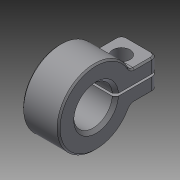
# Autodesk Inventor part: pipeClap
Saved by Autodesk Inventor 2014 SP1 (Build 180222100, 222)
## iProperties
Created: 2014-11-11
Part Number: pipeClap
Material: Generic
Document SubType Name: Modeling
Designer: rawrdong
Density: 1 g/cm^3
Appearance: Default
Author: rawrdong
Autodesk Inventor part; units mm, degrees
ref_plane "YZ Plane" through (0, 0, 0) normal (1, 0, 0) x (0, 1, 0)
ref_plane "XZ Plane" through (0, 0, 0) normal (0, 1, 0) x (-1, 0, 0)
ref_plane "XY Plane" through (0, 0, 0) normal (0, 0, 1) x (1, 0, 0)
sketch "Sketch1" plane through (0, 0, 0) normal (1, 0, 0) x (0, 1, 0)
  line L0 (0, 8.645) -> (0, -8.645) projected
  line L1 (-9.4444, 0) -> (13.4411, 0) projected
  circle A0 centre (0, 0) radius 6.175
  circle A1 centre (0, 0) radius 3.175
  line L2 (3.1687, -0.2) -> (6.1718, -0.2)
  line L3 (3.1687, 0.2) -> (6.1718, 0.2)
  line L4 (6.1718, 0.2) -> (10.1718, 0.2)
  line L5 (10.1718, 0.2) -> (10.1718, 2.45)
  line L6 (10.1718, 2.45) -> (5.6682, 2.45)
  line L7 (6.1718, -0.2) -> (10.1718, -0.2)
  line L8 (10.1718, -0.2) -> (10.1718, -2.45)
  line L9 (10.1718, -2.45) -> (5.6682, -2.45)
  dimension "d0" = 6.35
  dimension "d1" = 3
  dimension "d2" = 0.2
  dimension "d3" = 4
  dimension "d4" = 2.25
  constraints: 16 end point, 7 point on circle, 4 parallel, 2 centre point, 2 coincident, 2 perpendicular, 1 collinear, 1 point on line, 3 other
  measures "d0" diameter of A1
  measures "d1" radial gap between concentric circles of A0 A1
  measures "d2" distance between parallel lines of L3 L1
  measures "d3" distance of L7.start L7.end
  measures "d4" distance of L7.end L8.end
extrude "Extrusion1" add sketch "Sketch1" along normal blind 6 contours A0 L3 A1 L0 | L0 A1 L1 A0 | L6 L5 L4 A0 | L1 A1 L0 A0 | L0 A1 L2 A0 | A0 L7 L8 L9
sketch "Sketch2" plane through (0, 5.6682, -2.45) normal (0, 0, -1) x (-1, 0, 0)
  line L0 (0, 4.5036) -> (-6, 4.5036) projected
  circle A0 centre (-3, 1.5) radius 1.5
  circle A1 centre (-3, 1.5) radius 2.6 construction
  line L1 (0, 0) -> (-6, 0) projected
  point P0 (0, -5.6682)
  point P1 (-3, 4.5036)
  dimension "d8" = 3
  dimension "d24" = 5.2
  constraints: 2 centre point, 1 coincident, 1 midpoint, 1 tangent, 1 vertical alignment
  measures "d8" diameter of A0
  measures "d24" diameter of A1
extrude "Extrusion2" cut sketch "Sketch2" against normal up to surface (2.25 mm away)
sketch "Sketch4" plane through (0, 5.6682, 2.45) normal (0, 0, 1) x (1, 0, 0)
  circle A0 centre (3, 1.5) radius 1.5 projected
  circle A1 centre (3, 1.5) radius 1.5 projected
  circle A2 centre (3, 1.5) radius 1.425
  point P0 (0, -5.6682)
  point P1 (3, 0)
  dimension "d14" = 2.85
  constraints: 1 centre point, 1 coincident, 1 vertical alignment
  measures "d14" diameter of A2
extrude "Extrusion4" cut sketch "Sketch4" against normal through all contours A2
fillet "Fillet2" radius 1 7 edges at (6, 10.1718, 1.325) (3, 5.6682, 2.45) (0, 10.1718, 1.325) (0, 10.1718, -1.325) (6, 10.1718, -1.325) (1.5, 5.6682, -2.45) (4.5, 5.6682, -2.45)
chamfer "Chamfer1" distance 0.5 angle 45 2 edges at (6, -3.175, 0) (0, -3.175, 0)
sketch "Sketch5" plane through (0, 6.2911, -2.45) normal (0, 0, -1) x (-1, 0, 0)
  arc A0 (-1.7831, 0) -> (-4.2169, 0) centre (-3, 0.8771) ccw projected
  circle A1 centre (-3, 0.8771) radius 2.7
  circle A2 centre (-3, 0.8771) radius 1.5
  point P0 (0, -6.2911)
  dimension "d25" = 5.4
  constraints: 2 centre point, 2 coincident, 1 concentric
  measures "d25" diameter of A1
extrude "Extrusion5" cut sketch "Sketch5" along normal through all contours A2 A0 | A1
chamfer "Chamfer2" distance 0.25 angle 45 16 edges at (6, -6.175, 0) (6, 9.1718, -1.325) (6, 7.7314, -2.45) (5.7071, 9.8789, -2.45) (3, 10.1718, -2.45) (0.2929, 9.8789, -2.45) (0, 7.7314, -2.45) (0, 9.1718, -1.325) (0, -6.175, 0) (0, 9.1718, 1.325) (0, 7.7314, 2.45) (0.2929, 9.8789, 2.45) (3, 10.1718, 2.45) (5.7071, 9.8789, 2.45) (6, 7.7314, 2.45) (6, 9.1718, 1.325)
sketch "Sketch3" plane through (0, 5.6682, 2.45) normal (0, 0, 1) x (1, 0, 0)
  circle A0 centre (2.5, 3.2518) radius 1.5 projected
  circle A1 centre (2.5, 3.2518) radius 1.5 projected
  line L0 (4.3187, 6.4018) -> (6.1373, 3.2518)
  line L1 (6.1373, 3.2518) -> (4.3187, 0.1018)
  line L2 (4.3187, 0.1018) -> (0.6813, 0.1018)
  line L3 (0.6813, 0.1018) -> (-1.1373, 3.2518)
  line L4 (-1.1373, 3.2518) -> (0.6813, 6.4018)
  line L5 (0.6813, 6.4018) -> (4.3187, 6.4018)
  point P0 (0, -5.6682)
  dimension "d11" = 6.3
  constraints: 12 end point, 1 coincident, 1 horizontal, 13 other
  measures "d11" distance between parallel lines of L5 L2
body "Solid1"
